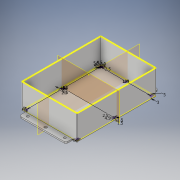
# Autodesk Inventor part: Main Enclosure Base 2
Saved by Autodesk Inventor 2019 (Build 230136000, 136)
## iProperties
Created: 2020-02-20
Part Number: Main Enclosure Base 2
Material: Generic
Document SubType Name: Modeling
Designer: gfb14170
Density: 1 g/cm^3
Appearance: Default
Author: gfb14170
Autodesk Inventor part; units mm, degrees
ref_plane "XZ Plane" through (0, 0, 0) normal (0, 1, 0) x (-1, 0, 0)
sketch "Sketch1" plane through (0, 0, 0) normal (0, 1, 0) x (-1, 0, 0)
  line L0 (60.4, 85.9) -> (-60.4, 85.9)
  line L1 (-60.4, 85.9) -> (-60.4, -85.9)
  line L2 (-60.4, -85.9) -> (60.4, -85.9)
  line L3 (60.4, -85.9) -> (60.4, 85.9)
  point P0 (0, 0)
  dimension "d0" = 85.9
  dimension "d1" = 85.9
  dimension "d2" = 60.4
  dimension "d3" = 60.4
  constraints: 8 end point, 2 parallel, 1 horizontal, 1 perpendicular
  measures "d0" distance from line of point (0, 0) L2
  measures "d1" distance from line of L0 point (0, 0)
  measures "d2" distance from line of point (0, 0) L3
  measures "d3" distance from line of L1 point (0, 0)
extrude "Extrusion1" add sketch "Sketch1" along normal blind 55.05
fillet "Fillet1" radius 2 6 edges at (60.4, 27.525, 85.9) (-60.4, 27.525, 85.9) (60.4, 27.525, -85.9) (-60.4, 27.525, -85.9) (60.4, 0, 0) (-60.4, 0, 0)
sketch "Sketch2" plane through (0, 55.05, 0) normal (0, 1, 0) x (1, 0, 0)
  line L0 (-58.4, -83.9) -> (58.4, -83.9)
  line L1 (58.4, -83.9) -> (58.4, 83.9)
  line L2 (58.4, 83.9) -> (-58.4, 83.9)
  line L3 (-58.4, 83.9) -> (-58.4, -83.9)
  line L4 (-60.4, 83.9) -> (-60.4, -83.9) projected
  line L5 (-58.4, -85.9) -> (58.4, -85.9) projected
  line L6 (60.4, -83.9) -> (60.4, 83.9) projected
  line L7 (58.4, 85.9) -> (-58.4, 85.9) projected
  point P0 (0, 0)
  dimension "d7" = 2
  dimension "d8" = 2
  dimension "d9" = 2
  dimension "d10" = 2
  constraints: 8 end point, 2 parallel, 1 horizontal, 1 perpendicular
  measures "d7" distance between parallel lines of L4 L3
  measures "d8" distance between parallel lines of L5 L0
  measures "d9" distance between parallel lines of L6 L1
  measures "d10" distance between parallel lines of L7 L2
extrude "Extrusion2" cut sketch "Sketch2" against normal blind 53.05
sketch "Sketch3" plane through (0, 0, 0) normal (0, -1, 0) x (1, 0, 0)
  line L0 (-58.4, -85.9) -> (-58.4, 85.9) projected
  line L1 (58.4, -85.9) -> (-58.4, -85.9) projected
  line L2 (58.4, 85.9) -> (58.4, -85.9) projected
  line L3 (-58.4, 85.9) -> (58.4, 85.9) projected
  line L4 (-58.4, 85.9) -> (58.4, 85.9) projected
  line L5 (50.4, 85.9) -> (50.4, 99.9)
  line L6 (50.4, 99.9) -> (-50.4, 99.9)
  line L7 (-50.4, 99.9) -> (-50.4, 85.9)
  line L8 (-60.4, 83.9) -> (-60.4, -83.9) projected
  line L9 (60.4, -83.9) -> (60.4, 83.9) projected
  line L10 (-134.6994, 0) -> (135.5184, 0) construction
  line L11 (50.4, -85.9) -> (50.4, -99.9)
  line L12 (50.4, -99.9) -> (-50.4, -99.9)
  line L13 (-50.4, -99.9) -> (-50.4, -85.9)
  line L14 (50.4, 85.9) -> (-50.4, 85.9)
  line L15 (-50.4, -85.9) -> (50.4, -85.9)
  point P0 (0, 0)
  dimension "d13" = 10
  dimension "d14" = 10
  dimension "d15" = 14
  dimension "d16" = 0
  constraints: 18 end point, 4 symmetric about line, 2 parallel, 1 collinear, 1 horizontal, 1 point on line
  measures "d13" distance between parallel lines of L8 L7
  measures "d14" distance between parallel lines of L5 L9
  measures "d15" distance between parallel lines of L3 L6
  measures "d16" distance from line of point (0, 0) L10
extrude "Extrusion3" add sketch "Sketch3" against normal blind 3 contours L1 L11 L12 L13 | L7 L6 L5 L3
fillet "Fillet2" radius 4 4 edges at (-50.4, 1.5, -99.9) (50.4, 1.5, -99.9) (50.4, 1.5, 99.9) (-50.4, 1.5, 99.9)
fillet "Fillet3" radius 2 8 edges at (-59.8142, 0.5858, 85.3142) (-54.4, 0, 85.9) (59.8142, 0.5858, 85.3142) (54.4, 0, 85.9) (59.8142, 0.5858, -85.3142) (54.4, 0, -85.9) (-59.8142, 0.5858, -85.3142) (-54.4, 0, -85.9)
sketch "Sketch4" plane through (0, 2, 0) normal (0, 1, 0) x (1, 0, 0)
  circle A0 centre (-54.9, 80.4) radius 1.25
  line L0 (58.4, 85.9) -> (-58.4, 85.9) projected
  line L1 (-60.4, 83.9) -> (-60.4, -83.9) projected
  circle A1 centre (54.1, 80.4) radius 1.25
  circle A2 centre (-54.9, -79.6) radius 1.25
  circle A3 centre (54.1, -79.6) radius 1.25
  circle A4 centre (-54.9, 80.4) radius 2.25
  circle A5 centre (-54.9, -79.6) radius 2.25
  circle A6 centre (54.1, 80.4) radius 2.25
  circle A7 centre (54.1, -79.6) radius 2.25
  line L2 (-58.4, 83.9) -> (-60.4, 83.9) projected
  line L3 (-58.4, 83.9) -> (-58.4, 75.9)
  line L4 (-58.4, 83.9) -> (-58.4, -83.9) projected
  line L5 (-58.4, 85.9) -> (-58.4, 83.9) projected
  line L6 (-58.4, 83.9) -> (-50.4, 83.9)
  line L7 (-58.4, 83.9) -> (58.4, 83.9) projected
  arc A8 (-55.4407, 78.2159) -> (-58.4, 75.9) centre (-56.0141, 75.9) ccw
  arc A9 (-50.4, 83.9) -> (-52.7159, 80.9407) centre (-50.4, 81.5141) ccw
  line L8 (58.4, 83.9) -> (58.4, -83.9) projected
  line L9 (58.4, 83.9) -> (48.8739, 83.9)
  line L10 (58.4, 83.9) -> (58.4, 75.9)
  line L11 (58.4, -83.9) -> (58.4, 83.9) projected
  line L12 (58.4, -83.9) -> (-58.4, -83.9) projected
  line L13 (-58.4, -83.9) -> (-58.4, -75.9)
  line L14 (-58.4, -83.9) -> (-58.4, 83.9) projected
  line L15 (-58.4, -83.9) -> (-50.4, -83.9)
  arc A10 (-52.7997, -80.4071) -> (-50.4, -83.9) centre (-50.4, -81.3292) ccw
  arc A11 (-58.4, -75.9) -> (-55.8323, -77.5522) centre (-56.5846, -75.9) ccw
  line L16 (58.4, -83.9) -> (50.4, -83.9)
  line L17 (58.4, -83.9) -> (58.4, -75.9)
  arc A12 (55.2614, -77.6729) -> (58.4, -75.9) centre (56.33, -75.9) ccw
  arc A13 (50.4, -83.9) -> (52.1729, -80.7614) centre (50.4, -81.83) ccw
  circle A14 centre (54.5, 0) radius 1.25
  circle A15 centre (-54.5, 0) radius 1.25
  circle A16 centre (-54.5, 0) radius 2.25
  circle A17 centre (54.5, 0) radius 2.25
  line L18 (54.5, -2.25) -> (56.9, -2.25)
  line L19 (54.5, 2.25) -> (56.9, 2.25)
  line L20 (-54.5, -2.25) -> (-56.9, -2.25)
  line L21 (-54.5, 2.25) -> (-56.9, 2.25)
  line L22 (0, 85.9) -> (0, 75.9)
  line L23 (-58.4, -83.9) -> (-58.4, 83.9) projected
  line L24 (58.4, -83.9) -> (-58.4, -83.9) projected
  line L25 (-58.4, 83.9) -> (58.4, 83.9) projected
  arc A18 (58.4, -3.75) -> (56.9, -2.25) centre (56.9, -3.75) ccw
  line L26 (58.4, 83.9) -> (58.4, -83.9) projected
  arc A19 (56.9, 2.25) -> (58.4, 3.75) centre (56.9, 3.75) ccw
  arc A20 (-56.9, -2.25) -> (-58.4, -3.75) centre (-56.9, -3.75) ccw
  arc A21 (-58.4, 3.75) -> (-56.9, 2.25) centre (-56.9, 3.75) ccw
  arc A22 (51.8602, 80.6143) -> (48.8739, 83.9) centre (48.8739, 80.9) ccw
  arc A23 (58.4, 75.3135) -> (54.6571, 78.2201) centre (55.4, 75.3135) ccw
  line L27 (-58.4, 75.9) -> (-58.4, 83.7116)
  line L28 (-58.4, 75.9) -> (-58.4, 83.9)
  line L29 (-50.4, 83.9) -> (-58.4, 83.9)
  line L30 (60.4, 83.9) -> (58.4, 83.9) projected
  line L31 (48.8739, 83.9) -> (58.4, 83.9)
  line L32 (58.4, 83.9) -> (58.4, 75.3135)
  point P0 (0, 0)
  point P1 (58.4, -2.25)
  point P2 (58.4, 2.25)
  point P3 (-58.4, -2.25)
  point P4 (-58.4, 2.25)
  dimension "d21" = 2.5
  dimension "d23" = 5.5
  dimension "d24" = 5.5
  dimension "d27" = 109
  dimension "d30" = 160
  dimension "d33" = 4.5
  dimension "d36" = 160
  dimension "d39" = 109
  dimension "d42" = 8
  dimension "d43" = 8
  dimension "d46" = 8
  dimension "d47" = 8
  dimension "d48" = 8
  dimension "d49" = 8
  dimension "d52" = 2.5
  dimension "d53" = 2.5
  dimension "d54" = 3.9
  dimension "d56" = 3.9
  dimension "d57" = 0
  dimension "d58" = 0
  dimension "d59" = 4.5
  dimension "d60" = 4.5
  dimension "d115" = 1.5
  dimension "d116" = 1.5
  dimension "d117" = 1.5
  dimension "d118" = 1.5
  dimension "d119" = 3
  dimension "d120" = 3
  constraints: 36 end point, 36 point on circle, 24 centre point, 21 tangent, 13 point on line, 4 horizontal, 3 coincident, 3 collinear, 3 perpendicular, 3 vertical, 1 midpoint, 27 other
  measures "d21" diameter of A0
  measures "d23" distance from line of L0 A0.centre
  measures "d24" distance from line of L1 A0.centre
  measures "d27" distance of A0.centre A1.centre
  measures "d30" distance of A0.centre A2.centre
  measures "d33" diameter of A4
  measures "d36" distance of A4.centre A5.centre
  measures "d39" distance of A4.centre A6.centre
  measures "d42" distance of L2.start L3.end
  measures "d43" distance of L2.start L6.end
  measures "d46" distance of L4.end L13.end
  measures "d47" distance of L4.end L15.end
  measures "d48" distance of L8.end L16.end
  measures "d49" distance of L8.end L17.end
  measures "d52" diameter of A14
  measures "d53" diameter of A15
  measures "d54" distance from line of A14.centre L8
  measures "d56" distance from line of A15.centre L14
  measures "d57" vertical distance of A14.centre point (0, 0)
  measures "d58" vertical distance of point (0, 0) A15.centre
  measures "d59" diameter of A16
  measures "d60" diameter of A17
  measures "d115" radius of A19
  measures "d116" radius of A18
  measures "d117" radius of A21
  measures "d118" radius of A20
  measures "d119" radius of A23
  measures "d120" radius of A22
sketch "Sketch6" plane through (0, 3, 0) normal (0, 1, 0) x (1, 0, 0)
  circle A0 centre (40.4, 92.9) radius 2.5
  line L0 (50.4, 85.9) -> (50.4, 95.9) projected
  line L1 (46.4, 99.9) -> (-46.4, 99.9) projected
  circle A1 centre (-39.6, 92.9) radius 2.5
  circle A2 centre (40.4, -92.1) radius 2.5
  circle A3 centre (-39.6, -92.1) radius 2.5
  circle A4 centre (0, 92.9) radius 3
  circle A5 centre (0, -92.9) radius 3
  line L2 (-50.4, -85.9) -> (50.4, -85.9) projected
  line L3 (0, 139.86) -> (0, -139.86) projected
  line L4 (50.4, 85.9) -> (-50.4, 85.9) projected
  point P0 (0, 0)
  dimension "d62" = 5
  dimension "d63" = 10
  dimension "d64" = 7
  dimension "d67" = 80
  dimension "d70" = 185
  dimension "d109" = 6
  dimension "d110" = 6
  dimension "d111" = 7
  dimension "d112" = 0
  dimension "d113" = 7
  dimension "d114" = 0
  constraints: 6 centre point, 1 horizontal, 1 vertical, 6 other
  measures "d62" diameter of A0
  measures "d63" distance from line of L0 A0.centre
  measures "d64" distance from line of L1 A0.centre
  measures "d67" distance of A0.centre A1.centre
  measures "d70" distance of A0.centre A2.centre
  measures "d109" diameter of A4
  measures "d110" diameter of A5
  measures "d111" distance from line of L2 A5.centre
  measures "d112" distance from line of L3 A5.centre
  measures "d113" distance from line of L4 A4.centre
  measures "d114" distance from line of L3 A4.centre
extrude "Extrusion5" cut sketch "Sketch6" against normal blind 3
sketch "Sketch8" plane through (0, 55.05, 0) normal (0, 1, 0) x (1, 0, 0)
  line L0 (58.4, 83.9) -> (58.4, -83.9) projected
  line L1 (58.4, -83.9) -> (-58.4, -83.9) projected
  line L2 (-58.4, -83.9) -> (-58.4, 83.9) projected
  line L3 (-58.4, 83.9) -> (58.4, 83.9) projected
  arc A0 (-60.4, -83.9) -> (-58.4, -85.9) centre (-58.4, -83.9) ccw projected
  line L4 (-58.4, -85.9) -> (58.4, -85.9) projected
  arc A1 (58.4, -85.9) -> (60.4, -83.9) centre (58.4, -83.9) ccw projected
  line L5 (60.4, -83.9) -> (60.4, 83.9) projected
  arc A2 (60.4, 83.9) -> (58.4, 85.9) centre (58.4, 83.9) ccw projected
  line L6 (58.4, 85.9) -> (-58.4, 85.9) projected
  arc A3 (-58.4, 85.9) -> (-60.4, 83.9) centre (-58.4, 83.9) ccw projected
  line L7 (-60.4, 83.9) -> (-60.4, -83.9) projected
  point P0 (0, 0)
equation "\"d1\" = d0"
equation "\"d3\" = d2"
equation "\"d7\" = d8"
equation "\"d9\" = d8"
equation "\"d10\" = d8"
body "Solid1"
